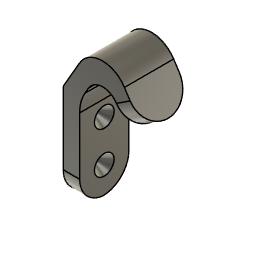
pieza 1 v1 (Autodesk Fusion 360 design; units mm, degrees)
Autodesk Fusion 360 part; units mm, degrees
note: some values were not read from the file. Chosen so that the rebuilt part matches the saved one: which face or edge a step refers to; which pieces of a blend or face edit are solid.
sketch "Boceto1" plane through (0, 0, 0) normal (0, 0, 1) x (1, 0, 0)
  line L0 (0, 0) -> (0, 30)
  line L1 (0, 0) -> (5.0043, -8.6677)
  line L2 (18.6509, -9.0109) -> (24.476, 0)
  line L3 (5, 1.3397) -> (5, 30)
  line L4 (5, 1.3397) -> (7.6988, -3.3347)
  line L5 (16.2279, -3.5491) -> (20.277, 2.7145)
  line L6 (5, 30) -> (0, 30)
  line L7 (24.476, 0) -> (20.277, 2.7145)
  arc A0 (7.6988, -3.3347) -> (16.2279, -3.5491) centre (12.0289, -0.8347) ccw
  arc A1 (5.0043, -8.6677) -> (18.6509, -9.0109) centre (11.9325, -4.6677) ccw
  point P0 (11.547, -20)
  dimension "d1" = 30
  dimension "d2" = 20
  dimension "d3" = 150
  dimension "d5" = 20
  dimension "d6" = 5
  dimension "d7" = 8
  constraint vertical L0
  constraint coincident L0.start L1.start
  constraint perpendicular L0 L6
  constraint perpendicular L2 L7
  constraint tangent L4 A0
  constraint tangent L5 A0
  constraint coincident P0 L1
  constraint coincident P0 L2
  constraint tangent L1 A1
  constraint tangent L2 A1
  measures "d1" distance of L0.start L0.end
  measures "d2" vertical distance of L0.start P0
  measures "d3" angle of L0 L1
  measures "d5" vertical distance of P0 L2.end
  measures "d6" radius of A0
  measures "d7" radius of A1
extrude "Extruir1" add sketch "Boceto1" along normal blind 15
sketch "Boceto2" plane through (5, 0, 0) normal (1, 0, 0) x (0, 1, 0)
  line L0 (1.3397, 0) -> (30, 0)
  line L1 (30, 0) -> (30, 15)
  line L2 (30, 15) -> (1.3397, 15)
  line L3 (1.3397, 15) -> (1.3397, 0)
  line L4 (15.6699, 15) -> (15.6699, 0) construction
  line L5 (30, 7.5) -> (1.3397, 7.5) construction
  circle A0 centre (9.3397, 7.5) radius 3
  circle A1 centre (22, 7.5) radius 3
  dimension "d10" = 6
  dimension "d11" = 8
  constraint midpoint L2 L4.start
  constraint midpoint L0 L4.end
  constraint midpoint L1 L5.start
  constraint midpoint L3 L5.end
  constraint coincident L5 A0.centre
  constraint symmetric L4 A0 A1
  measures "d10" diameter of A0
  measures "d11" distance of L5.end A0.centre
extrude "Extruir2" cut sketch "Boceto2" against normal blind 3 draft -35 contours A0 | A1
extrude "Extruir3" cut 2 faces at (2, 9.6098, 7.3699) (2, 21.3767, 7.4369) along direction (-1, 0, 0) through all
fillet "Empalme1" radius 7.5 3 edges at (22.3765, 1.3572, 15) (20.277, 2.7145, 7.5) (22.3765, 1.3572, 0)
fillet "Empalme2" radius 8 4 edges at (0, 30, 7.5) (2.5, 30, 0) (2.5, 30, 15) (5, 30, 7.5)
fillet "Empalme3" radius 12 1 edges at (5, 1.3397, 7.5)
move_body "Desplazar1" bodies 1 to x (1, 0, 0) y (0, 0, -1) z (0, 1, 0) at (0, 13.3089, 13.3089)
